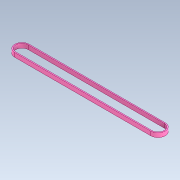
# Autodesk Inventor part: elastico
Saved by Autodesk Inventor 2022 (Build 260153000, 153)
## iProperties
Created: 2022-11-16
Part Number: elastico
Material: Generic
Document SubType Name: Modeling
Designer: ferna
Density: 1 g/cm^3
Appearance: Pink
Author: ferna
Autodesk Inventor part; units mm, degrees
ref_plane "YZ Plane" through (0, 0, 0) normal (1, 0, 0) x (0, 1, 0)
ref_plane "XZ Plane" through (0, 0, 0) normal (0, 1, 0) x (-1, 0, 0)
ref_plane "XY Plane" through (0, 0, 0) normal (0, 0, 1) x (1, 0, 0)
sketch "Sketch1" plane through (0, 0, 0) normal (0, 1, 0) x (-1, 0, 0)
  circle A0 centre (0, 0) radius 1.5
  line L0 (0, 0) -> (33.03, 0)
  circle A1 centre (33.03, 0) radius 1.5
  circle A2 centre (33.03, 0) radius 1.75
  circle A3 centre (0, 0) radius 1.75
  line L1 (33.03, 1.75) -> (0, 1.75)
  line L2 (0, -1.75) -> (33.03, -1.75)
  line L3 (33.03, -1.5) -> (0, -1.5)
  line L4 (0, 1.5) -> (33.03, 1.5)
  dimension "d0" = 3
  dimension "d1" = 33.03
  dimension "d2" = 3
  dimension "d3" = 3.5
  constraints: 10 end point, 8 point on circle, 6 tangent, 4 centre point, 4 coincident, 1 horizontal
  measures "d0" diameter of A0
  measures "d1" distance of L0.start L0.end
  measures "d2" diameter of A1
  measures "d3" diameter of A2
extrude "Extrusion1" add sketch "Sketch1" along normal blind 1 contours A0 L3 A3 L4 | A3 L1 A2 L4 | L3 A2 L2 A3 | A2 L3 A1 L4
body "Solid1"
